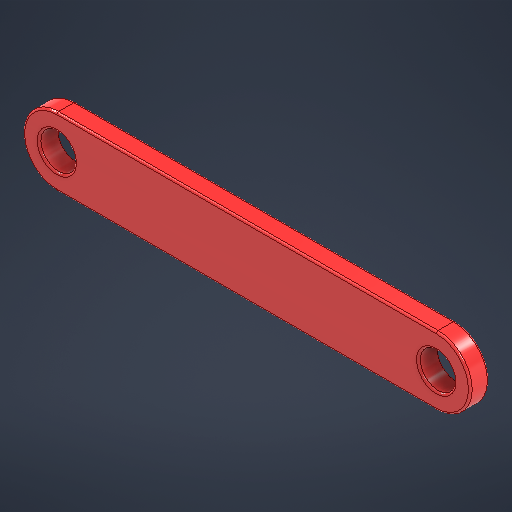
# Autodesk Inventor part: Arm Link Cross
Saved by Autodesk Inventor 2026.2 (Build 302298010, 298A)
## iProperties
Created: 2026-05-28
Part Number: Arm Link Cross
Material: Generic
Document SubType Name: Modeling
Designer: yassi
Density: 1 g/cm^3
Appearance: Light Red
Author: yassi
Autodesk Inventor part; units mm, degrees
ref_plane "YZ Plane" through (0, 0, 0) normal (1, 0, 0) x (0, 1, 0)
ref_plane "XZ Plane" through (0, 0, 0) normal (0, 1, 0) x (-1, 0, 0)
ref_plane "XY Plane" through (0, 0, 0) normal (0, 0, 1) x (1, 0, 0)
sketch "Sketch1" plane through (0, 0, 0) normal (0, 0, 1) x (1, 0, 0)
  circle A0 centre (0, 0) radius 4.7
  circle A1 centre (100, 0) radius 4.7
  circle A2 centre (0, 0) radius 9
  circle A3 centre (100, 0) radius 9
  line L0 (0, 9) -> (100, 9)
  line L1 (0, -9) -> (100, -9)
  dimension "d0" = 9.4
  dimension "d2" = 9.4
  dimension "d3" = 18
  dimension "d4" = 18
  constraints: 4 centre point, 4 end point, 4 point on circle, 3 coincident, 1 horizontal, 1 parallel, 1 tangent
  measures "d0" diameter of A0
  measures "d2" diameter of A1
  measures "d3" diameter of A2
  measures "d4" diameter of A3
extrude "Extrusion1" add sketch "Sketch1" along normal blind 5
fillet "Fillet1" radius 0.5 8 edges at (50, -9, 5) (109, 0, 5) (50, 9, 5) (-9, 0, 5) (50, -9, 0) (109, 0, 0) (50, 9, 0) (-9, 0, 0)
fillet "Fillet2" radius 0.5 2 edges at (-4.7, 0, 5) (95.3, 0, 5)
body "Solid1"
